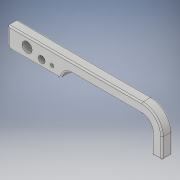
# Autodesk Inventor part: BRAZO BALSA UNDIMOTRIZ
Saved by Autodesk Inventor 2019.4 (Build 234330000, 330)
## iProperties
Created: 2020-08-23
Part Number: BRAZO BALSA UNDIMOTRIZ
Material: Generic
Document SubType Name: Modeling
Designer: crist
Density: 1 g/cm^3
Appearance: Default
Author: crist
Autodesk Inventor part; units mm, degrees
ref_plane "YZ Plane" through (0, 0, 0) normal (1, 0, 0) x (0, 1, 0)
ref_plane "XZ Plane" through (0, 0, 0) normal (0, 1, 0) x (-1, 0, 0)
ref_plane "XY Plane" through (0, 0, 0) normal (0, 0, 1) x (1, 0, 0)
sketch "Boceto1" plane through (0, 0, 0) normal (0, 0, 1) x (1, 0, 0)
  arc A0 (1500, 0) -> (0, 1500) centre (0, 0) ccw
  arc A1 (3000, 0) -> (0, 3000) centre (0, 0) ccw
  line L0 (3000, 0) -> (3000, -3000)
  line L1 (3000, -3000) -> (1500, -3000)
  line L2 (1500, -3000) -> (1500, 0)
  line L3 (0, 3000) -> (-20000, 3000)
  line L4 (-20000, 3000) -> (-20000, 0)
  line L5 (-20000, 0) -> (-12000, 0)
  arc A2 (-10500, 1500) -> (-12000, 0) centre (-10500, 0) ccw
  line L6 (0, 1500) -> (-10500, 1500)
  dimension "d4" = 3000
  dimension "d5" = 6000
  dimension "d7" = 20000
  dimension "d8" = 8000
  dimension "d10" = 3000
  constraints: 14 end point, 6 point on circle, 4 perpendicular, 3 centre point, 2 coincident, 2 horizontal, 1 vertical
  measures "d4" diameter of A0
  measures "d5" diameter of A1
  measures "d7" distance of L3.start L3.end
  measures "d8" distance of L4.end L5.end
  measures "d10" distance of L0.start L0.end
extrude "Extrusión1" add sketch "Boceto1" along normal blind 1500
fillet "Empalme1" radius 500 1 edges at (-12000, 0, 750)
sketch "Boceto2" plane through (0, 0, 1500) normal (0, 0, 1) x (1, 0, 0)
  circle A0 centre (-13410.7545, 1088.9074) radius 250
  circle A1 centre (-14953.0607, 1088.9074) radius 500
  circle A2 centre (-17138.5672, 1588.9074) radius 750
  point P0 (0, 0)
  dimension "d14" = 500
  dimension "d15" = 1000
  dimension "d16" = 1500
  constraints: 3 centre point
  measures "d14" diameter of A0
  measures "d15" diameter of A1
  measures "d16" diameter of A2
extrude "Extrusión2" cut sketch "Boceto2" against normal blind 1500
fillet "Empalme2" radius 500 1 edges at (-20000, 0, 750)
fillet "Empalme3" radius 200 1 edges at (2250, -3000, 1500)
fillet "Empalme4" radius 200 1 edges at (2250, -3000, 0)
fillet "Empalme5" radius 200 28 edges at (3000, -2941.4214, 1441.4214) (3000, -1400, 1500) (2121.3203, 2121.3203, 1500) (-10000, 3000, 1500) (3000, -2941.4214, 58.5786) (3000, -1400, 0) (2121.3203, 2121.3203, 0) (-10000, 3000, 0) (3000, -3000, 750) (1500, -2941.4214, 1441.4214) (1500, -1400, 1500) (1060.6602, 1060.6602, 1500) (-5250, 1500, 1500) (-11418.5587, 1185.8541, 1500) (-12130.3055, 104.7153, 1500) (-15968.2458, 0, 1500) (-19853.5534, 146.4466, 1500) (-20000, 1750, 1500) (1500, -2941.4214, 58.5786) (1500, -1400, 0) (1060.6602, 1060.6602, 0) (-5250, 1500, 0) (-11418.5587, 1185.8541, 0) (-12130.3055, 104.7153, 0) (-15968.2458, 0, 0) (-19853.5534, 146.4466, 0) (-20000, 1750, 0) (1500, -3000, 750)
